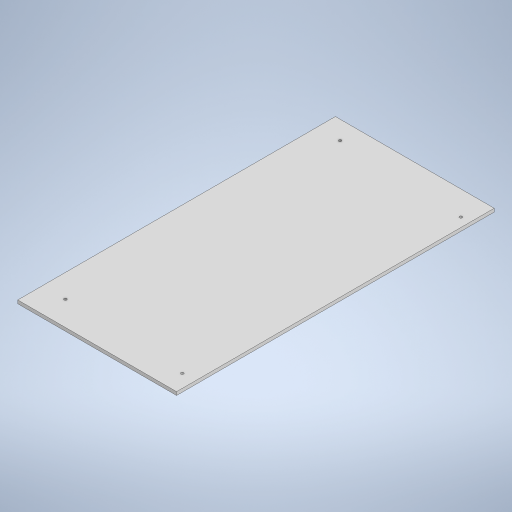
# Autodesk Inventor part: OdorMachineShelf
Saved by Autodesk Inventor 2023 (Build 270158000, 158)
## iProperties
Created: 2023-06-14
Part Number: OdorMachineShelf
Material: Generic
Document SubType Name: Modeling
Designer: User
Density: 1 g/cm^3
Appearance: Default
Author: User
Autodesk Inventor part; units mm, degrees
ref_plane "YZ Plane" through (0, 0, 0) normal (1, 0, 0) x (0, 1, 0)
ref_plane "XZ Plane" through (0, 0, 0) normal (0, 1, 0) x (-1, 0, 0)
ref_plane "XY Plane" through (0, 0, 0) normal (0, 0, 1) x (1, 0, 0)
sketch "Sketch1" plane through (0, 0, 0) normal (0, 1, 0) x (-1, 0, 0)
  line L0 (-152.4, 304.8) -> (152.4, 304.8)
  line L1 (152.4, 304.8) -> (152.4, -304.8)
  line L2 (152.4, -304.8) -> (-152.4, -304.8)
  line L3 (-152.4, -304.8) -> (-152.4, 304.8)
  line L4 (-152.4, 304.8) -> (152.4, -304.8) construction
  line L5 (152.4, 304.8) -> (-152.4, -304.8) construction
  point P0 (0, 0)
  dimension "d0" = 609.6
  dimension "d1" = 304.8
  constraints: 12 end point, 2 midpoint, 2 parallel, 1 horizontal, 1 perpendicular
  measures "d0" distance of L0.end L1.end
  measures "d1" distance of L1.end L2.end
extrude "Extrusion1" add sketch "Sketch1" along normal blind 6.35
sketch "Sketch2" plane through (0, 6.35, 0) normal (0, 1, 0) x (1, 0, 0)
  circle A0 centre (-107.95, 269.24) radius 2.54
  circle A1 centre (134.9375, 258.1275) radius 2.54
  line L0 (152.4, 304.8) -> (-152.4, 304.8) projected
  line L1 (-152.4, 304.8) -> (-152.4, -304.8) projected
  circle A2 centre (-107.95, -257.81) radius 2.54
  circle A3 centre (127.3548, -268.9352) radius 2.54
  point P0 (0, 0)
  dimension "d4" = 242.8875
  dimension "d8" = 44.45
  dimension "d9" = 11.1252
  dimension "d10" = 527.05
  dimension "d11" = 5.08
  dimension "d12" = 5.08
  dimension "d13" = 5.08
  dimension "d14" = 5.08
  dimension "d15" = 11.1125
  dimension "d16" = 35.56
  constraints: 4 centre point
  measures "d4" horizontal distance of A1.centre A0.centre
  measures "d8" distance from line of L1 A0.centre
  measures "d9" vertical distance of A3.centre A2.centre
  measures "d10" distance of A0.centre A2.centre
  measures "d11" diameter of A0
  measures "d12" diameter of A1
  measures "d13" diameter of A2
  measures "d14" diameter of A3
  measures "d15" vertical distance of A1.centre A0.centre
  measures "d16" distance from line of L0 A0.centre
extrude "Extrusion2" cut sketch "Sketch2" against normal up to next
body "Solid1"
